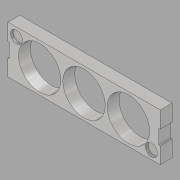
# Autodesk Inventor part: Tube Holder
Saved by Autodesk Inventor 2017 (Build 210142000, 142)
## iProperties
Created: 2016-12-06
Part Number: Tube Holder
Material: Aluminum 6061-AHC
Document SubType Name: Modeling
Designer: qupec
Density: 2.7 g/cm^3
Appearance: Aluminum - Dark
Mass: 20.4912 g
Surface Area: 43.8677 cm^2
Volume: 7.58934 cm^3
Author: qupec
Autodesk Inventor part; units mm, degrees
ref_plane "YZ Plane" through (0, 0, 0) normal (1, 0, 0) x (0, 1, 0)
ref_plane "XZ Plane" through (0, 0, 0) normal (0, 1, 0) x (-1, 0, 0)
ref_plane "XY Plane" through (0, 0, 0) normal (0, 0, 1) x (1, 0, 0)
sketch "Sketch1" plane through (0, 0, 0) normal (0, 0, 1) x (1, 0, 0)
  line L0 (-40.64, 12.7) -> (40.64, 12.7)
  line L1 (40.64, 12.7) -> (40.64, -12.7)
  line L2 (40.64, -12.7) -> (-40.64, -12.7)
  line L3 (-40.64, -12.7) -> (-40.64, 12.7)
  point P0 (0, 0)
  dimension "d0" = 81.28
  dimension "d1" = 40.64
  dimension "d2" = 12.7
  dimension "d3" = 25.4
  constraints: 8 end point, 2 parallel, 1 horizontal, 1 perpendicular
  measures "d0" distance of L0.start L0.end
  measures "d1" distance from line of point (0, 0) L3
  measures "d2" distance from line of point (0, 0) L2
  measures "d3" distance of L2.end L0.start
extrude "Extrusion1" add sketch "Sketch1" along normal mid plane 6.35
sketch "Sketch2" plane through (0, 0, 3.175) normal (0, 0, 1) x (1, 0, 0)
  circle A0 centre (-23.7067, 0) radius 11.303
  circle A1 centre (0, 0) radius 11.303
  line L0 (40.64, -12.7) -> (40.64, 12.7) projected
  circle A2 centre (23.7067, 0) radius 11.303
  line L1 (-40.64, 12.7) -> (-40.64, -12.7) projected
  line L2 (-40.64, 0) -> (40.64, 0) construction
  line L3 (40.64, 12.7) -> (-40.64, 12.7) projected
  point P0 (0, 0)
  dimension "d6" = 22.606
  dimension "d9" = 22.606
  dimension "d11" = 22.606
  dimension "d14" = 23.7067
  dimension "d21" = 81.28
  dimension "d22" = 23.7067
  dimension "d45" = 0
  constraints: 3 centre point, 3 midpoint, 2 end point, 1 point on line
  measures "d6" diameter of A0
  measures "d9" diameter of A1
  measures "d11" diameter of A2
  measures "d14" distance of A1.centre A0.centre
  measures "d21" distance of L0.end L1.start
  measures "d22" distance of A2.centre A1.centre
  measures "d45" distance of point (0, 0) A1.centre
sketch "Sketch4" plane through (-40.64, -12.7, -3.175) normal (-1, 0, 0) x (0, 0, 1)
  line L0 (0, 0) -> (0, 25.4) projected
  line L1 (6.35, 25.4) -> (6.35, 0) projected
  line L2 (0, 16.51) -> (6.35, 16.51)
  line L3 (6.35, 16.51) -> (6.35, 8.89)
  line L4 (6.35, 8.89) -> (0, 8.89)
  line L5 (0, 8.89) -> (0, 16.51)
  point P0 (3.175, 12.7)
  point P1 (0, 25.4)
  dimension "d30" = 3.81
  dimension "d31" = 7.62
  constraints: 8 end point, 2 parallel, 1 horizontal, 1 perpendicular, 1 point on line, 2 other
  measures "d30" distance from line of point (3.175, 12.7) L4
  measures "d31" distance between parallel lines of L4 L2
extrude "Extrusion3" cut sketch "Sketch4" against normal blind 0.635
mirror "Mirror1" about plane through (0, 0, 0) normal (1, 0, 0) of "Extrusion3"
sketch "Sketch5" plane through (0, 0, 3.175) normal (0, 0, 1) x (1, 0, 0)
  circle A0 centre (0, 8.128) radius 3.175 construction
  line L0 (40.64, 12.7) -> (-40.64, 12.7) projected
  line L1 (-22.0846, 0) -> (40.005, 0) construction
  line L2 (40.005, 3.81) -> (40.005, -3.81) projected
  circle A1 centre (0, -8.128) radius 3.175 construction
  circle A2 centre (-36.068, 8.128) radius 3.175
  circle A3 centre (36.068, -8.128) radius 3.175
  line L3 (-40.64, 12.7) -> (-40.64, 3.81) projected
  line L4 (40.64, -3.81) -> (40.64, -12.7) projected
  line L5 (40.64, -12.7) -> (-40.64, -12.7) projected
  point P0 (0, 0)
  dimension "d34" = 6.35
  dimension "d35" = 4.572
  dimension "d48" = 6.35
  dimension "d49" = 6.35
  dimension "d50" = 4.572
  dimension "d51" = 4.572
  dimension "d52" = 4.572
  dimension "d53" = 4.572
  constraints: 4 centre point, 2 end point, 1 midpoint, 1 symmetric about line, 1 other
  measures "d34" diameter of A0
  measures "d35" distance from line of L0 A0.centre
  measures "d48" diameter of A2
  measures "d49" diameter of A3
  measures "d50" distance from line of L0 A2.centre
  measures "d51" distance from line of L3 A2.centre
  measures "d52" distance from line of L4 A3.centre
  measures "d53" distance from line of L5 A3.centre
extrude "Extrusion4" cut sketch "Sketch5" against normal blind 1.27
sketch "Sketch7" plane through (-40.64, -12.7, 3.175) normal (0, -1, 0) x (1, 0, 0)
  line L0 (26.67, -14.605) -> (54.61, -14.605)
  line L1 (54.61, -14.605) -> (54.61, 8.255)
  line L2 (54.61, 8.255) -> (26.67, 8.255)
  line L3 (26.67, 8.255) -> (26.67, -14.605)
  point P0 (40.64, -3.175)
  dimension "d39" = 27.94
  dimension "d40" = 22.86
  dimension "d41" = 11.43
  dimension "d42" = 13.97
  constraints: 8 end point, 2 parallel, 1 horizontal, 1 perpendicular
  measures "d39" distance of L0.start L0.end
  measures "d40" distance of L2.end L0.start
  measures "d41" distance from line of point (40.64, -3.175) L0
  measures "d42" distance from line of point (40.64, -3.175) L1
extrude "Extrusion5" [suppressed]
extrude "Extrusion6" cut sketch "Sketch2" against normal blind 25.4
sketch "Sketch8" plane through (0, 0, -3.175) normal (0, 0, -1) x (-1, 0, 0)
  line L0 (40.005, 3.81) -> (40.005, -3.81) construction
  line L1 (40.005, 0) -> (-40.005, 0)
  line L2 (-40.005, 3.81) -> (-40.005, -3.81) construction
  line L3 (40.64, 12.7) -> (-40.64, 12.7) projected
  line L4 (40.64, 3.81) -> (40.64, 12.7) projected
  line L5 (-40.64, 12.7) -> (-40.64, 3.81) projected
  line L6 (-40.005, 3.81) -> (-40.005, 0)
  line L7 (-40.64, 3.81) -> (-40.005, 3.81) projected
  line L8 (40.005, 3.81) -> (40.005, 0)
  line L9 (40.005, 3.81) -> (40.64, 3.81) projected
  point P0 (0, 0)
  constraints: 6 end point, 2 collinear, 2 midpoint
extrude "Extrusion7" [suppressed]
sketch "Sketch9" plane through (0, 0, -3.175) normal (0, 0, -1) x (-1, 0, 0)
  line L0 (-40.64, -12.7) -> (40.64, -12.7) projected
  line L1 (40.64, -12.7) -> (40.64, -3.81) projected
  line L2 (40.64, -3.81) -> (40.005, -3.81) projected
  line L3 (-40.005, -3.81) -> (-40.64, -3.81) projected
  line L4 (-40.64, -3.81) -> (-40.64, -12.7) projected
  line L5 (-40.005, 3.81) -> (-40.005, -3.81) projected
  line L6 (-40.005, 0) -> (-40.005, -3.81)
  line L7 (-40.005, 0) -> (40.005, 0)
  line L8 (40.005, -3.81) -> (40.005, 3.81) projected
  line L9 (40.005, -3.81) -> (40.005, 0)
  point P0 (0, 0)
  constraints: 6 end point, 2 collinear, 2 midpoint
extrude "Extrusion8" [suppressed]
equation "\"d1\" = 0.5 * d0"
equation "\"d2\" = 0.5 * d3"
equation "\"d9\" = d7"
equation "\"d11\" = d9"
equation "\"d22\" = d14"
equation "\"d30\" = 0.5 * d31"
equation "\"d41\" = 0.5 * d40"
equation "\"d42\" = 0.5 * d39"
equation "\"d7\" = d6"
body "Solid1"
